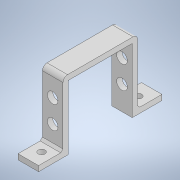
# Autodesk Inventor part: Stepper Motor Mount
Saved by Autodesk Inventor 2021 (Build 250183000, 183)
## iProperties
Created: 2021-06-25
Part Number: Stepper Motor Mount
Material: Generic
Document SubType Name: Modeling
Designer: Work
Density: 1 g/cm^3
Appearance: Default
Author: Work
Autodesk Inventor part; units mm, degrees
ref_plane "YZ Plane" through (0, 0, 0) normal (1, 0, 0) x (0, 1, 0)
ref_plane "XZ Plane" through (0, 0, 0) normal (0, 1, 0) x (-1, 0, 0)
ref_plane "XY Plane" through (0, 0, 0) normal (0, 0, 1) x (1, 0, 0)
sketch "Sketch1" plane through (0, 0, 0) normal (1, 0, 0) x (0, 1, 0)
  line L0 (0, -25) -> (42.2, -25)
  line L1 (3.5, -21.5) -> (45.7, -21.5)
  line L2 (42.2, -25) -> (42.2, -67)
  line L3 (45.7, -21.5) -> (45.7, -70.5)
  line L4 (42.2, -67) -> (3.5, -67)
  line L5 (45.7, -70.5) -> (3.5, -70.5)
  line L6 (3.5, -67) -> (0, -67)
  line L7 (3.5, -21.5) -> (3.5, -5.5)
  line L8 (3.5, -5.5) -> (0, -5.5)
  line L9 (0, -5.5) -> (0, -25)
  line L10 (3.5, -70.5) -> (3.5, -86.5)
  line L11 (3.5, -86.5) -> (0, -86.5)
  line L12 (0, -86.5) -> (0, -67)
  point P0 (0, 0)
  dimension "d3" = 42.2
  dimension "d4" = 42
  dimension "d5" = 3.5
  dimension "d7" = 3.5
  dimension "d19" = 16
  dimension "d20" = 16
  constraints: 26 end point, 5 horizontal, 5 vertical, 3 perpendicular
  measures "d3" distance of L0.start L0.end
  measures "d4" distance of L0.end L2.end
  measures "d5" distance between parallel lines of L2 L3
  measures "d7" distance between parallel lines of L4 L5
  measures "d19" distance of L1.start L7.end
  measures "d20" distance of L5.end L10.end
extrude "Extrusion1" add sketch "Sketch1" against normal blind 13.5
sketch "Sketch3" plane through (0, 3.5, -5.5) normal (0, 1, 0) x (1, 0, 0)
  circle A0 centre (-6.75, 8.75) radius 2.25
  circle A1 centre (-6.75, 72.25) radius 2.25
  line L0 (0, 16) -> (0, 0) projected
  line L1 (0, 81) -> (0, 65) projected
  line L2 (0, 0) -> (-13.5, 0) projected
  line L3 (0, 81) -> (-13.5, 81) projected
  point P0 (0, -5.5)
  dimension "d21" = 4.5
  dimension "d22" = 4.5
  dimension "d23" = 6.75
  dimension "d24" = 6.75
  dimension "d25" = 8.75
  dimension "d26" = 8.75
  constraints: 2 centre point
  measures "d21" diameter of A0
  measures "d22" diameter of A1
  measures "d23" distance from line of L0 A0.centre
  measures "d24" distance from line of L1 A1.centre
  measures "d25" distance from line of L2 A0.centre
  measures "d26" distance from line of L3 A1.centre
extrude "Extrusion3" cut sketch "Sketch3" against normal through all
fillet "Fillet1" radius 3 2 edges at (-6.75, 45.7, -21.5) (-6.75, 45.7, -70.5)
chamfer "Chamfer1" distance 1.5 angle 45 2 edges at (-6.75, 3.5, -21.5) (-6.75, 3.5, -70.5)
sketch "Sketch5" plane through (0, 42.7, -70.5) normal (0, 0, -1) x (-1, 0, 0)
  circle A0 centre (6.75, -12) radius 3.5
  line L0 (13.5, 3) -> (0, 3) projected
  line L1 (13.5, 0) -> (13.5, -37.7) projected
  point P0 (0, -42.7)
  dimension "d44" = 7
  dimension "d45" = 15
  dimension "d51" = 6.75
  constraints: 1 centre point
  measures "d44" diameter of A0
  measures "d45" distance from line of A0.centre L0
  measures "d51" distance from line of L1 A0.centre
extrude "Extrusion5" cut sketch "Sketch5" against normal through all
pattern_linear "Rectangular Pattern2" count 2 spacing 15 along (0, -1, 0) of "Extrusion5"
body "Solid1"
